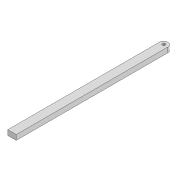
# Autodesk Inventor part: Part_10_p2
Saved by Autodesk Inventor 2022 (Build 260153000, 153)
## iProperties
Created: 2022-04-22
Part Number: Part_10_p2
Material: Generic
Document SubType Name: Modeling
Designer: dell
Density: 1 g/cm^3
Appearance: Default
Mass: 4.34309 g
Surface Area: 38.0975 cm^2
Volume: 4.34309 cm^3
Author: dell
Autodesk Inventor part; units mm, degrees
ref_plane "YZ Plane" through (0, 0, 0) normal (1, 0, 0) x (0, 1, 0)
ref_plane "XZ Plane" through (0, 0, 0) normal (0, 1, 0) x (-1, 0, 0)
ref_plane "XY Plane" through (0, 0, 0) normal (0, 0, 1) x (1, 0, 0)
sketch "Sketch1" plane through (0, 0, 0) normal (0, 1, 0) x (-1, 0, 0)
  line L0 (0, 0) -> (0, -355.998) construction
  line L1 (5, 0) -> (5, -355.998)
  line L2 (-5, -355.998) -> (-5, 0)
  arc A0 (5, 0) -> (-5, 0) centre (0, 0) ccw
  arc A1 (-5, -355.998) -> (5, -355.998) centre (0, -355.998) ccw
  circle A2 centre (0, 0) radius 1.65
  circle A3 centre (0, -355.998) radius 1.65
  circle A4 centre (0, -57.376) radius 1.65
  point P0 (0, -177.999)
  dimension "d0" = 3.3
  dimension "d1" = 3.3
  dimension "d2" = 10
  dimension "d3" = 355.998
  dimension "d14" = 3.3
  dimension "d15" = 57.376
  constraints: 8 end point, 5 centre point, 4 point on circle, 4 tangent, 2 coincident, 1 midpoint, 1 parallel, 1 point on line, 1 vertical
  measures "d0" diameter of A2
  measures "d1" diameter of A3
  measures "d2" distance between parallel lines of L2 L1
  measures "d3" distance of L0.end L0.start
  measures "d14" diameter of A4
  measures "d15" distance of L0.start A4.centre
extrude "Extrusion1" add sketch "Sketch1" along normal blind 6
sketch "Sketch2" plane through (0, 6, 0) normal (0, 1, 0) x (1, 0, 0)
  line L0 (-26.2185, 378.6248) -> (37.2853, 378.6248)
  line L1 (37.2853, 378.6248) -> (37.2853, 176.2061)
  line L2 (37.2853, 176.2061) -> (-26.2185, 176.2061)
  line L3 (-26.2185, 176.2061) -> (-26.2185, 378.6248)
  line L4 (-95.1798, 405.4155) -> (74.9908, 405.4155)
  line L5 (74.9908, 405.4155) -> (74.9908, -44.073)
  line L6 (74.9908, -44.073) -> (-95.1798, -44.073)
  line L7 (-95.1798, -44.073) -> (-95.1798, 405.4155)
  point P0 (0, 0)
  constraints: 16 end point, 4 parallel, 2 horizontal, 2 perpendicular
extrude "Extrusion2" cut sketch "Sketch2" against normal blind 10
body "Solid1"
